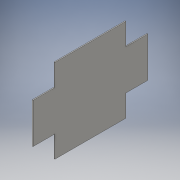
# Autodesk Inventor part: Bottom Plywood Piece
Saved by Autodesk Inventor 2016 SP2 (Build 200236200, 236)
## iProperties
Created: 2018-01-17
Part Number: Bottom Plywood Piece
Material: Generic
Document SubType Name: Modeling
Designer: CAD
Density: 1 g/cm^3
Appearance: Default
Author: CAD
Autodesk Inventor part; units mm, degrees
ref_plane "YZ Plane" through (0, 0, 0) normal (1, 0, 0) x (0, 1, 0)
ref_plane "XZ Plane" through (0, 0, 0) normal (0, 1, 0) x (-1, 0, 0)
ref_plane "XY Plane" through (0, 0, 0) normal (0, 0, 1) x (1, 0, 0)
sketch "Sketch1" plane through (0, 0, 0) normal (1, 0, 0) x (0, 1, 0)
  line L0 (0, 0) -> (-279.4, 0)
  line L1 (-279.4, 0) -> (-279.4, -152.4)
  line L2 (-279.4, -152.4) -> (-431.8, -152.4)
  line L3 (-431.8, -152.4) -> (-431.8, -647.7)
  line L4 (-431.8, -647.7) -> (-279.4, -647.7)
  line L5 (-279.4, -647.7) -> (-279.4, -800.1)
  line L6 (-279.4, -800.1) -> (0, -800.1)
  line L7 (0, -800.1) -> (0, -647.7)
  line L8 (0, -647.7) -> (152.4, -647.7)
  line L9 (152.4, -647.7) -> (152.4, -152.4)
  line L10 (152.4, -152.4) -> (0, -152.4)
  line L11 (0, 0) -> (0, -152.4)
  dimension "d0" = 279.4
  dimension "d1" = 152.4
  dimension "d2" = 152.4
  dimension "d3" = 495.3
  dimension "d4" = 152.4
  dimension "d5" = 152.4
  dimension "d6" = 279.4
  dimension "d7" = 152.4
  dimension "d8" = 152.4
  dimension "d9" = 495.3
  constraints: 24 end point, 7 point on line, 5 perpendicular, 1 horizontal
  measures "d0" distance of L0.start L0.end
  measures "d1" distance of L0.end L1.end
  measures "d2" distance of L1.end L2.end
  measures "d3" distance of L2.end L3.end
  measures "d4" distance of L3.end L4.end
  measures "d5" distance of L4.end L5.end
  measures "d6" distance of L5.end L6.end
  measures "d7" distance of L6.end L7.end
  measures "d8" distance of L7.end L8.end
  measures "d9" distance of L8.end L9.end
extrude "Extrusion1" add sketch "Sketch1" along normal blind 6.35
body "Solid1"
